Autodesk Fusion 360 part; units mm, degrees
(part 5 of 5)
sketch "スケッチ1 (6)" plane through (0, 0, 0) normal (0, 0, 1) x (1, 0, 0)
  line L0 (112.7582, 64.032, -12) -> (187.9303, 64.032, -12)
  line L1 (-187.9318, -64.0321, -12) -> (-197.3819, -54.5822, -12)
  line L2 (37.5852, -64.0321, -12) -> (-37.5867, -64.0321, -12)
  line L3 (112.7582, -64.0321, -12) -> (37.5852, -64.0321, -12)
  line L4 (197.3815, 18.1941, -12) -> (197.3815, -18.1937, -12)
  line L5 (-197.3819, -18.1941, -12) -> (-197.3819, 18.1941, -12)
  line L6 (-197.3819, 54.5821, -12) -> (-196.2819, 62.9319, -12)
  line L7 (197.3815, 54.5821, -12) -> (197.3815, 18.1941, -12)
  line L8 (187.9303, 64.032, -12) -> (196.2815, 62.9319, -12)
  line L9 (-187.9318, 64.032, -12) -> (-112.7598, 64.032, -12)
  line L10 (-112.7598, -64.0321, -12) -> (-187.9318, -64.0321, -12)
  line L11 (-112.7598, 64.032, -12) -> (-37.5867, 64.032, -12)
  line L12 (37.5855, 64.032, -12) -> (112.7582, 64.032, -12)
  line L13 (196.2815, 62.9319, -12) -> (197.3815, 54.5821, -12)
  line L14 (-197.3819, -54.5822, -12) -> (-197.3819, -18.1941, -12)
  line L15 (-37.5867, -64.0321, -12) -> (-112.7598, -64.0321, -12)
  line L16 (-196.2819, 62.9319, -12) -> (-187.9318, 64.032, -12)
  line L17 (197.3815, -54.5822, -12) -> (187.9303, -64.0321, -12)
  line L18 (187.9303, -64.0321, -12) -> (112.7582, -64.0321, -12)
  line L19 (-37.5867, 64.032, -12) -> (37.5855, 64.032, -12)
  line L20 (197.3815, -18.1937, -12) -> (197.3815, -54.5822, -12)
  line L21 (-197.3819, 18.1941, -12) -> (-197.3819, 54.5821, -12)
sketch "スケッチ2 (2)" plane through (0, 0, 0) normal (0, 0, 1) x (1, 0, 0)
  line L0 (-23.1948, 64.032, -12) -> (8.9054, 64.032, -12)
  line L1 (8.9054, 64.032, -12) -> (8.9054, 10.069, -12)
  line L2 (-23.1948, 10.069, -12) -> (-23.1948, 64.032, -12)
  line L3 (8.9054, 10.069, -12) -> (-23.1948, 10.069, -12)
sketch "スケッチ3 (2)" plane through (0, 0, 0) normal (0, 0, 1) x (1, 0, 0)
  line L0 (8.9054, 64.032, -16) -> (8.9054, 10.069, -16)
  line L1 (-23.1948, 10.069, -16) -> (-23.1948, 64.032, -16)
  line L2 (-23.1948, 64.032, -16) -> (8.9054, 64.032, -16)
  line L3 (8.9054, 10.069, -16) -> (-23.1948, 10.069, -16)
hole "穴1" at (196.2815, 62.9319, -12) at (-196.2819, 62.9319, -12) direction (0, 0, 1) diameter 4.234 depth 13 tip angle 180 bodies 4 in component "CaseBottom"
thread "ねじ1" "ISO Metric profile 5.0 M5x0.8 6H" major diameter 5.12 minor diameter 4.234 pitch 0.8 angle 60 resizes the face on face at (-197.8691, 64.3327, -8) on face at (197.294, 61.0728, -8) on bodies 4 in component "CaseBottom"
hole "穴2" at (187.9303, 64.032, -12) at (112.7582, 64.032, -12) at (37.5855, 64.032, -12) at (-37.5867, 64.032, -12) at (-112.7598, 64.032, -12) at (-187.9318, 64.032, -12) at (-197.3819, 54.5821, -12) at (-197.3819, 18.1941, -12) at (-197.3819, -18.1941, -12) at (-197.3819, -54.5822, -12) at (-187.9318, -64.0321, -12) at (-112.7598, -64.0321, -12) at (-37.5867, -64.0321, -12) at (37.5852, -64.0321, -12) at (112.7582, -64.0321, -12) at (187.9303, -64.0321, -12) at (197.3815, -54.5822, -12) at (197.3815, -18.1937, -12) at (197.3815, 18.1941, -12) at (197.3815, 54.5821, -12) direction (0, 0, 1) diameter 3 depth 19 tip angle 180 counterbore diameter 5.6 counterbore depth 2.1 bodies 4 in component "CaseBottom"
hole "穴1'" at (187.9303, 64.032, -12) at (112.7582, 64.032, -12) at (37.5855, 64.032, -12) at (-37.5867, 64.032, -12) at (-112.7598, 64.032, -12) at (-187.9318, 64.032, -12) at (-197.3819, 54.5821, -12) at (-197.3819, 18.1941, -12) at (-197.3819, -18.1941, -12) at (-197.3819, -54.5822, -12) at (-187.9318, -64.0321, -12) at (-112.7598, -64.0321, -12) at (-37.5867, -64.0321, -12) at (37.5852, -64.0321, -12) at (112.7582, -64.0321, -12) at (187.9303, -64.0321, -12) at (197.3815, -54.5822, -12) at (197.3815, -18.1937, -12) at (197.3815, 18.1941, -12) at (197.3815, 54.5821, -12) direction (0, 0, 1) diameter 3 depth 19 tip angle 180 counterbore diameter 5.6 counterbore depth 2.1 bodies 1 in component "CasePlateDefault"
hole "穴1''" at (187.9303, 64.032, -12) at (112.7582, 64.032, -12) at (37.5855, 64.032, -12) at (-37.5867, 64.032, -12) at (-112.7598, 64.032, -12) at (-187.9318, 64.032, -12) at (-197.3819, 54.5821, -12) at (-197.3819, 18.1941, -12) at (-197.3819, -18.1941, -12) at (-197.3819, -54.5822, -12) at (-187.9318, -64.0321, -12) at (-112.7598, -64.0321, -12) at (-37.5867, -64.0321, -12) at (37.5852, -64.0321, -12) at (112.7582, -64.0321, -12) at (187.9303, -64.0321, -12) at (197.3815, -54.5822, -12) at (197.3815, -18.1937, -12) at (197.3815, 18.1941, -12) at (197.3815, 54.5821, -12) direction (0, 0, 1) diameter 3 depth 19 tip angle 180 counterbore diameter 5.6 counterbore depth 2.1 bodies 2 in component "CasePlateExtended"
hole "穴1'''" at (187.9303, 64.032, -12) at (112.7582, 64.032, -12) at (37.5855, 64.032, -12) at (-37.5867, 64.032, -12) at (-112.7598, 64.032, -12) at (-187.9318, 64.032, -12) at (-197.3819, 54.5821, -12) at (-197.3819, 18.1941, -12) at (-197.3819, -18.1941, -12) at (-197.3819, -54.5822, -12) at (-187.9318, -64.0321, -12) at (-112.7598, -64.0321, -12) at (-37.5867, -64.0321, -12) at (37.5852, -64.0321, -12) at (112.7582, -64.0321, -12) at (187.9303, -64.0321, -12) at (197.3815, -54.5822, -12) at (197.3815, -18.1937, -12) at (197.3815, 18.1941, -12) at (197.3815, 54.5821, -12) direction (0, 0, 1) diameter 2.529 depth 19 tip angle 180 counterbore diameter 5.6 counterbore depth 2.1 bodies 3 in component "CaseTop"
thread "ねじ1'" "ISO Metric profile 3.0 M3x0.5 6H" major diameter 3.086 minor diameter 2.529 pitch 0.5 angle 60 resizes the face on face at (113.0088, 65.2714, 3.6667) on face at (36.3399, -64.2517, 3.6667) on face at (-112.5092, -62.7927, 3.6667) on face at (-38.8414, 64.1892, 3.6667) on face at (186.9822, -63.1954, 3.6667) on face at (-198.33, -53.7455, 3.6667) on face at (-196.4338, 17.3574, 3.6667) on face at (-112.5092, 65.2714, 3.6667) on face at (198.1943, -19.1624, 3.6667) on face at (196.4334, 55.4188, 3.6667) on face at (196.4334, -53.7455, 3.6667) on face at (36.3308, 64.1892, 3.6667) on face at (-38.832, -64.2517, 3.6667) on face at (186.9822, 64.8687, 3.6667) on face at (113.0088, -62.7927, 3.6667) on face at (198.3296, 17.3574, 3.6667) on face at (-188.8799, 64.8687, 3.6667) on face at (-196.4338, -19.0308, 3.6667) on face at (-198.33, 55.4188, 3.6667) on face at (-188.8799, -63.1954, 3.6667) on bodies 3 in component "CaseTop"
hole "穴1''''" at (8.9054, 64.032, -16) at (-23.1948, 64.032, -16) at (-23.1948, 10.069, -16) at (8.9054, 10.069, -16) direction (0, 0, 1) diameter 3 depth 3 tip angle 180 bodies 7 in component "CaseBottomPlate"
hole "穴3" at (8.9054, 64.032, -12) at (-23.1948, 64.032, -12) at (-23.1948, 10.069, -12) at (8.9054, 10.069, -12) direction (0, 0, 1) diameter 2.529 depth 9 tip angle 180 counterbore diameter 6.05 counterbore depth 1 bodies 4 in component "CaseBottom"
thread "ねじ2" "ISO Metric profile 3.0 M3x0.5 6H" major diameter 3.086 minor diameter 2.529 pitch 0.5 angle 60 resizes the face on face at (-23.0689, 11.3272, -9.6667) on face at (-24.4495, 64.1892, -8.3333) on face at (7.6507, 64.1892, -8.3333) on face at (9.0313, 11.3272, -9.6667) on bodies 4 in component "CaseBottom"
fillet "フィレット1" radius 1.5 4 edges at (-193.8817, 60.5321, -4.5) (193.8817, 60.5321, -4.5) (193.8817, -60.5321, -4.5) (-193.8817, -60.5321, -4.5) on bodies 4 in component "CaseBottom"
fillet "フィレット1" radius 2 2 edges at (-19.1949, 14.0689, -10.5) (4.9053, 14.0689, -10.5) on bodies 4 in component "CaseBottom"
fillet "フィレット1" radius 3 4 edges at (-201.3816, 68.0319, -6) (201.3816, 68.0319, -6) (201.3816, -68.0319, -6) (-201.3816, -68.0319, -6) on bodies 4 in component "CaseBottom"
fillet "フィレット1'" radius 1.5 18 edges at (-174.3318, 60.0319, 6) (-193.3816, 40.9808, 6) (-193.3816, 17.169, 6) (-93.3697, 60.0319, 6) (-93.3697, 36.2187, 6) (-174.3318, 40.9808, 6) (-193.3816, 20.9307, 6) (-193.3816, -60.0322, 6) (-93.3697, -60.0322, 6) (-97.1316, -60.0322, 6) (193.3816, -60.0322, 6) (193.3816, 39.9807, 6) (-97.1318, 20.9307, 6) (193.3816, 36.2187, 6) (193.3816, 60.0319, 6) (-97.1318, 17.169, 6) (-97.1316, 60.0319, 6) (-93.3697, 39.9807, 6) on bodies 3 in component "CaseTop"
fillet "フィレット1'" radius 3 4 edges at (-201.3816, 68.0317, 6) (-201.3816, -68.0317, 6) (201.3818, 68.0317, 6) (201.3818, -68.0317, 6) on bodies 3 in component "CaseTop"
chamfer "面取り1" distance 0.5 angle 45 9 edges at (0, -68.0319, 0) (-200.503, -67.1532, 0) (-201.3816, 0, 0) (-200.503, 67.1532, 0) (-108.7883, 68.0319, 0) (101.6435, 68.0319, 0) (200.503, 67.1532, 0) (201.3816, 0, 0) (200.503, -67.1532, 0) on bodies 4 in component "CaseBottom"
chamfer "面取り1" distance 0.809 angle 45 9 edges at (0, -68.0319, -12) (-200.503, -67.1532, -12) (-201.3816, 0, -12) (-200.503, 67.1532, -12) (-108.7883, 68.0319, -12) (101.6435, 68.0319, -12) (200.503, 67.1532, -12) (201.3816, 0, -12) (200.503, -67.1532, -12) on bodies 4 in component "CaseBottom"
chamfer "面取り1'" distance 0.5 angle 45 8 edges at (0.0001, -68.0317, 2) (200.5031, -67.153, 2) (201.3818, 0, 2) (200.5031, 67.153, 2) (0.0001, 68.0317, 2) (-200.503, 67.153, 2) (-201.3816, 0, 2) (-200.503, -67.153, 2) on bodies 3 in component "CaseTop"
chamfer "面取り1'" distance 0.809 angle 45 8 edges at (0.0001, -68.0317, 10) (200.5031, -67.153, 10) (201.3818, 0, 10) (200.5031, 67.153, 10) (0.0001, 68.0317, 10) (-200.503, 67.153, 10) (-201.3816, 0, 10) (-200.503, -67.153, 10) on bodies 3 in component "CaseTop"
component "CaseBottom" placed x (1, 0, 0) y (0, 1, 0) z (0, 0, 1) at (0, 0, 0)
component "CaseBottomPlate" placed x (1, 0, 0) y (0, 1, 0) z (0, 0, 1) at (0, 0, 0)
component "CaseTop" placed x (1, 0, 0) y (0, 1, 0) z (0, 0, 1) at (0, 0, 0)
component "CasePlateDefault" placed x (1, 0, 0) y (0, 1, 0) z (0, 0, 1) at (0, 0, 0)
component "CasePlateExtended" placed x (1, 0, 0) y (0, 1, 0) z (0, 0, 1) at (0, 0, 0)
